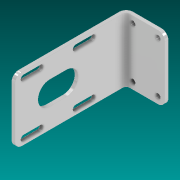
# Autodesk Inventor part: steppermount
Saved by Autodesk Inventor 2020.3 (Build 243373000, 373)
## iProperties
Created: 2020-05-24
Part Number: steppermount
Material: Aluminum 6061
Document SubType Name: Sheet Metal
Designer: Svend
Mass: 5.66404 g
Surface Area: 65.4079 cm^2
Volume: 5.66404 cm^3
Density: 2.7 g/cm^3
Sheet Metal Rule: Default_mm
Appearance: Aluminum - Polished
Author: Svend
Autodesk Inventor part; units mm, degrees
ref_plane "YZ Plane" through (0, 0, 0) normal (1, 0, 0) x (0, 1, 0)
ref_plane "XZ Plane" through (0, 0, 0) normal (0, 1, 0) x (-1, 0, 0)
ref_plane "XY Plane" through (0, 0, 0) normal (0, 0, 1) x (1, 0, 0)
ref_plane "Work Plane1" through (0, 0, 0) normal (0, 0, 1) x (1, 0, 0)
ref_plane "Work Plane2" through (0, 0, 0) normal (0, 0, 1) x (1, 0, 0)
sketch "Sketch4" plane through (0, 0, 0) normal (0, 0, 1) x (1, 0, 0)
  circle A0 centre (-15.9281, -36) radius 1.5
  circle A1 centre (-15.9281, -6) radius 1.5
  line L0 (-0.2416, -30) -> (0, -30)
  circle A2 centre (-1, -36) radius 1.5
  circle A3 centre (-0.9999, -6) radius 1.5
  circle A4 centre (-15.9281, -36) radius 1.5
  circle A5 centre (-15.928, -6) radius 1.5
  line L1 (6.7584, -40) -> (-19.9281, -40)
  line L2 (6.7584, -40) -> (6.7584, -30)
  line L3 (6.7584, -30) -> (7, -30.0001)
  line L4 (7.0001, -5.0001) -> (7, -30.0001)
  spline S0 degree 3 poles (8.2169, -2.0001) (8.1499, -2.073) (8.0847, -2.1482) (7.7881, -2.5121) (7.5886, -2.8263) (7.3052, -3.4054) (7.1888, -3.7186) (7.0362, -4.3634) (7.0001, -4.6952) (7.0001, -5.0001) knots 0 0 0 0 0.087816 0.087816 0.414412 0.414412 0.707206 0.707206 1 1 1 1
  line L5 (-19.928, -2) -> (8.2169, -2.0001)
  line L6 (-19.9281, -40) -> (-19.928, -2)
  line L7 (-19.928, -2) -> (3.072, -2)
  line L8 (3.072, -2) -> (3.072, -40)
  line L9 (3.072, -40) -> (-19.928, -40)
  line L10 (-19.928, -40) -> (-19.928, -2)
  point P0 (0, 0)
  dimension "d43" = 23
  measures "d43" distance of L8.end L9.end
extrude "Plate3" add sketch "Sketch4" along normal blind 2 contours L1 L6 L5 L8
sketch "Sketch5" plane through (-19.9281, -40, 2) normal (-1, 0.0000034, 0) x (-0.0000034, -1, 0)
  line L0 (-38, 0) -> (0, 0)
  line L1 (0, 0) -> (0, 66)
  line L2 (0, 66) -> (-38, 66)
  line L3 (-38, 66) -> (-38, 0)
  constraints: 6 end point, 1 horizontal, 1 perpendicular, 1 vertical
edge flange "Flange2" height 68 angle 90 thickness 2 bend radius 2 thickness toward (-1, 0.0000034, 0) relief straight relief width 2 relief depth 1 edges at (-19.9281, -21, 2) wall of the first edge with corners at (-19.928, -2, 2) (-19.9281, -40, 2) (-19.9281, -40, 68) (-19.928, -2, 68)
bend "Bend2"
corner "Corner2"
sketch "Sketch7" plane through (-21.9281, -40, 4) normal (-1, 0.0000034, 0) x (0, 0, 1)
  line L0 (17.9786, 3.5) -> (27.9786, 3.5) construction
  line L1 (17.9786, 1.75) -> (27.9786, 1.75)
  line L2 (27.9786, 5.25) -> (17.9786, 5.25)
  arc A0 (17.9786, 5.25) -> (17.9786, 1.75) centre (17.9786, 3.5) ccw
  arc A1 (27.9786, 1.75) -> (27.9786, 5.25) centre (27.9786, 3.5) ccw
  line L3 (17.9786, 34.5) -> (27.9786, 34.5) construction
  line L4 (17.9786, 32.75) -> (27.9786, 32.75)
  line L5 (27.9786, 36.25) -> (17.9786, 36.25)
  arc A2 (17.9786, 36.25) -> (17.9786, 32.75) centre (17.9786, 34.5) ccw
  arc A3 (27.9786, 32.75) -> (27.9786, 36.25) centre (27.9786, 34.5) ccw
  line L6 (48.9786, 34.5) -> (58.9786, 34.5) construction
  line L7 (48.9786, 32.75) -> (58.9786, 32.75)
  line L8 (58.9786, 36.25) -> (48.9786, 36.25)
  arc A4 (48.9786, 36.25) -> (48.9786, 32.75) centre (48.9786, 34.5) ccw
  arc A5 (58.9786, 32.75) -> (58.9786, 36.25) centre (58.9786, 34.5) ccw
  line L9 (48.9786, 3.5) -> (58.9786, 3.5) construction
  line L10 (48.9786, 1.75) -> (58.9786, 1.75)
  line L11 (58.9786, 5.25) -> (48.9786, 5.25)
  arc A6 (48.9786, 5.25) -> (48.9786, 1.75) centre (48.9786, 3.5) ccw
  arc A7 (58.9786, 1.75) -> (58.9786, 5.25) centre (58.9786, 3.5) ccw
  line L12 (33.4786, 19) -> (43.4786, 19) construction
  line L13 (33.4786, 13) -> (43.4786, 13)
  line L14 (43.4786, 25) -> (33.4786, 25)
  arc A8 (33.4786, 25) -> (33.4786, 13) centre (33.4786, 19) ccw
  arc A9 (43.4786, 13) -> (43.4786, 25) centre (43.4786, 19) ccw
  line L15 (33.4786, 12) -> (43.4786, 12)
  arc A10 (43.4786, 12) -> (43.4786, 26) centre (43.4786, 19) ccw
  line L16 (43.4786, 26) -> (33.4786, 26)
  arc A11 (33.4786, 26) -> (33.4786, 12) centre (33.4786, 19) ccw
  ellipse E0 centre (51.0785, 24.0319) end of major axis (51.3495, 30.0258) minor radius 0 projected
  ellipse E1 centre (50.628, 39.5682) end of major axis (50.7071, 41.3164) minor radius 0 projected
  ellipse E2 centre (49.2282, 8.5997) end of major axis (49.3072, 10.3479) minor radius 0 projected
  ellipse E3 centre (48.6301, 39.6584) end of major axis (48.7091, 41.4066) minor radius 0 projected
  ellipse E4 centre (49.2282, 8.5998) end of major axis (49.3072, 10.348) minor radius 0 projected
  point P0 (-4, 40)
  dimension "d49" = 1
  constraints: 44 end point, 24 point on circle, 20 tangent, 12 centre point, 7 parallel, 3 horizontal, 1 point on line, 8 other
  measures "d49" radial gap between concentric circles of A8 A11
extrude "Cut3" cut sketch "Sketch7" against normal blind 2 contours A0 L2 A1 L1 | A2 L5 A3 L4 | A4 L8 A5 L7 | A6 L11 A7 L10 | A8 L14 A9 L13 | A11 L16 A10 L15
fillet "Corner Round3" radius 4 4 edges at (3.072, -2, 1) (3.072, -40, 1) (-20.928, -2, 68) (-20.9281, -40, 68)
equation "\"d50\" = Thickness"
equation "\"d21\" = Thickness"
equation "\"d22\" = BendReliefWidth"
equation "\"d23\" = BendReliefDepth"
equation "\"d24\" = MinimumRemnant"
equation "\"d25\" = TransitionRadius"
equation "\"d28\" = BendRadius"
equation "\"d29\" = CornerReliefSize"
equation "\"d30\" = GapSize"
equation "\"d31\" = JacobiRadiusSize"
equation "\"BendRadius\" = Thickness"
equation "\"BendReliefWidth\" = Thickness"
equation "\"BendReliefDepth\" = 0.5 * Thickness"
equation "\"CornerReliefSize\" = 4 * Thickness"
equation "\"MinimumRemnant\" = 2 * Thickness"
equation "\"TransitionRadius\" = BendRadius"
equation "\"JacobiRadiusSize\" = BendRadius"
equation "\"GapSize\" = Thickness"
equation "\"Thickness\" = 2"
body "Solid2"
